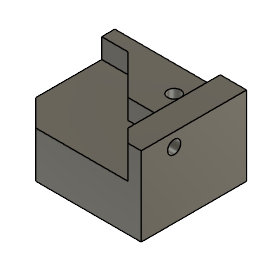
RoboconT1(Part-1) (Autodesk Fusion 360 design; units mm, degrees)
part number: 2026-03-05-11-02-33-637
Autodesk Fusion 360 part; units mm, degrees
sketch "Sketch1" plane through (0, 0, 0) normal (0, 0, 1) x (1, 0, 0)
  line L0 (50, 40) -> (-50, 40)
  line L1 (-50, 40) -> (-50, -20)
  line L2 (-30, -40) -> (50, -40)
  line L3 (50, -40) -> (50, 40)
  line L4 (-50, -20) -> (-30, -40)
  line L5 (-50, 40) -> (-50, 30)
  line L6 (-50, 30) -> (-30, 30)
  line L7 (-30, 30) -> (0, 0)
  line L8 (30, 0) -> (30, 40)
  line L9 (30, -30) -> (40, -40)
  line L10 (30, 0) -> (30, -30)
  line L11 (0, 0) -> (30, 0)
  constraint horizontal L0
  constraint perpendicular L0 L1
  constraint parallel L0 L2
  constraint parallel L1 L3
  constraint coincident L7.end L11.start
  constraint perpendicular L0 L5
  constraint perpendicular L5 L6
  constraint coincident L0 L8.end
  constraint perpendicular L0 L8
  constraint perpendicular L8 L11
extrude "Extrude1" add sketch "Sketch1" along normal blind 60 contours L0 L2 L3 L8 L9 L10
extrude "Extrude2" add sketch "Sketch1" along normal blind 50 contours L0 L1 L5 L6 L7 L8 L11
extrude "Extrude3" add sketch "Sketch1" along normal blind 35 contours L1 L2 L4 L6 L7 L9 L10 L11
sketch "Sketch4" plane through (0, 0, 50) normal (0, 0, 1) x (-1, 0, 0)
  line L0 (0, 0) -> (-30, 0)
  line L1 (-30, 0) -> (-30, -40)
  line L2 (-30, -40) -> (50, -40)
  line L3 (50, -40) -> (50, -30)
  line L4 (50, -30) -> (30, -30)
  line L5 (30, -30) -> (0, 0)
  circle A0 centre (-15, -20) radius 5
sketch "Sketch5" plane through (30, 0, 0) normal (-1, 0, 0) x (0, -1, 0)
  line L0 (0, 35) -> (30, 35)
  line L1 (30, 35) -> (30, 60)
  line L2 (30, 60) -> (-40, 60)
  line L3 (-40, 60) -> (-40, 50)
  line L4 (-40, 50) -> (0, 50)
  line L5 (0, 50) -> (0, 35)
  circle A0 centre (15, 50) radius 5
extrude "Extrude4" cut sketch "Sketch4" against normal blind 50 contours A0
extrude "Extrude5" cut sketch "Sketch5" against normal blind 20 contours A0
